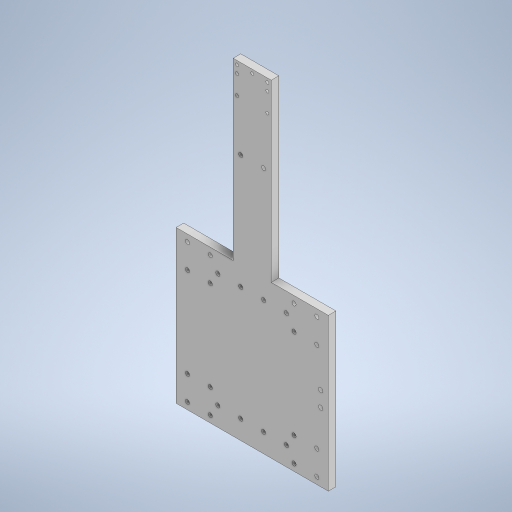
# Autodesk Inventor part: base sotto
Saved by Autodesk Inventor 2024 (Build 280153000, 153)
## iProperties
Created: 2023-12-23
Part Number: base sotto
Material: Generico
Document SubType Name: Modeling
Designer: Giorgio
Density: 1 g/cm^3
Appearance: Default
Mass: 400 g
Surface Area: 880 cm^2
Volume: 400 cm^3
Author: Giorgio
Autodesk Inventor part; units mm, degrees
ref_plane "YZ Plane" through (0, 0, 0) normal (1, 0, 0) x (0, 1, 0)
ref_plane "XZ Plane" through (0, 0, 0) normal (0, 1, 0) x (-1, 0, 0)
ref_plane "XY Plane" through (0, 0, 0) normal (0, 0, 1) x (1, 0, 0)
sketch "Schizzo1" plane through (0, 0, 0) normal (0, 0, 1) x (1, 0, 0)
  line L0 (100, 100) -> (-100, 100)
  line L1 (-100, 100) -> (-100, -100)
  line L2 (-100, -100) -> (100, -100)
  line L3 (100, -100) -> (100, 100)
  line L4 (25, 330) -> (-25, 330)
  line L5 (-25, 330) -> (-25, 100)
  line L6 (-25, 100) -> (25, 100)
  line L7 (25, 100) -> (25, 330)
  circle A0 centre (-20, 325) radius 2
  circle A1 centre (20, 325) radius 2
  circle A2 centre (0, 325) radius 2
  circle A3 centre (85, 91) radius 2.75
  circle A4 centre (85, 59) radius 2.75
  circle A5 centre (55, 91) radius 2.75
  circle A6 centre (55, 59) radius 2.75
  circle A7 centre (85, -59) radius 2.75
  circle A8 centre (-55, -59) radius 2.75
  circle A9 centre (-55, 91) radius 2.75
  circle A10 centre (85, -91) radius 2.75
  circle A11 centre (55, -59) radius 2.75
  circle A12 centre (55, -91) radius 2.75
  circle A13 centre (-85, 91) radius 2.75
  circle A14 centre (-55, 59) radius 2.75
  circle A15 centre (-85, 59) radius 2.75
  circle A16 centre (-85, -59) radius 2.75
  circle A17 centre (-55, -91) radius 2.75
  circle A18 centre (-85, -91) radius 2.75
  circle A19 centre (45, 75) radius 2.75
  circle A20 centre (45, -75) radius 2.75
  circle A21 centre (-45, -75) radius 2.75
  circle A22 centre (-45, 75) radius 2.75
  circle A23 centre (15, 75) radius 2.75
  circle A24 centre (15, -75) radius 2.75
  circle A25 centre (-15, -75) radius 2.75
  circle A26 centre (-15, 75) radius 2.75
  circle A27 centre (15, 225) radius 2.75
  circle A28 centre (-15, 225) radius 2.75
  circle A29 centre (20, 315) radius 2
  circle A30 centre (-20, 315) radius 2
  circle A31 centre (20, 290) radius 2
  circle A32 centre (-20, 290) radius 2
  circle A33 centre (90, 10) radius 3
  circle A34 centre (90, -10) radius 3
  point P0 (0, 0)
  point P1 (25, 100)
  point P2 (0, -100)
  dimension "d0" = 200
  dimension "d1" = 200
  dimension "d4" = 230
  dimension "d5" = 50
  dimension "d6" = 75
  dimension "d7" = 0
  dimension "d8" = 0
  dimension "d9" = 4
  dimension "d10" = 4
  dimension "d11" = 4
  dimension "d12" = 5
  dimension "d13" = 40
  dimension "d14" = 20
  dimension "d15" = 5
  dimension "d16" = 100
  dimension "d17" = 100
  dimension "d18" = 5.5
  dimension "d21" = 32
  dimension "d24" = 30
  dimension "d27" = 5.5
  dimension "d28" = 5.5
  dimension "d29" = 5.5
  dimension "d32" = 32
  dimension "d35" = 30
  dimension "d40" = 30
  dimension "d43" = 32
  dimension "d48" = 30
  dimension "d51" = 32
  dimension "d54" = 150
  dimension "d55" = 59
  dimension "d56" = 150
  dimension "d57" = 59
  dimension "d58" = 15
  dimension "d59" = 15
  dimension "d60" = 15
  dimension "d61" = 15
  dimension "d62" = 5.5
  dimension "d63" = 5.5
  dimension "d64" = 5.5
  dimension "d65" = 5.5
  dimension "d66" = 5.5
  dimension "d67" = 5.5
  dimension "d68" = 5.5
  dimension "d69" = 5.5
  dimension "d70" = 30
  dimension "d71" = 30
  dimension "d72" = 0
  dimension "d73" = 30
  dimension "d74" = 30
  dimension "d75" = 0
  dimension "d76" = 150
  dimension "d77" = 75
  dimension "d79" = 15
  dimension "d80" = 0
  dimension "d81" = 0
  dimension "d82" = 30
  dimension "d83" = 0
  dimension "d84" = 5.5
  dimension "d85" = 5.5
  dimension "d86" = 0
  dimension "d87" = 0
  dimension "d88" = 150
  dimension "d89" = 0
  dimension "d90" = 4
  constraints: 35 centre point, 16 end point, 6 horizontal, 5 vertical, 4 parallel, 2 perpendicular, 1 midpoint, 1 point on line, 26 other
  measures "d0" distance of L2.end L0.start
  measures "d1" distance of L0.start L0.end
  measures "d4" distance of L6.end L4.start
  measures "d5" distance of L4.start L4.end
  measures "d6" distance between parallel lines of L3 L7
  measures "d7" vertical distance of A1.centre A2.centre
  measures "d8" vertical distance of A2.centre A0.centre
  measures "d9" diameter of A0
  measures "d10" diameter of A2
  measures "d11" diameter of A1
  measures "d12" distance from line of L4 A1.centre
  measures "d13" distance of A0.centre A1.centre
  measures "d14" distance of A1.centre A2.centre
  measures "d15" distance from line of L7 A1.centre
  measures "d16" distance from line of L1 point (0, 0)
  measures "d17" distance of point (0, -100) point (0, 0)
  measures "d18" diameter of A3
  measures "d21" distance of A3.centre A4.centre
  measures "d24" distance of A3.centre A5.centre
  measures "d27" diameter of A7
  measures "d28" diameter of A8
  measures "d29" diameter of A9
  measures "d32" distance of A7.centre A10.centre
  measures "d35" distance of A7.centre A11.centre
  measures "d40" distance of A9.centre A13.centre
  measures "d43" distance of A9.centre A14.centre
  measures "d48" distance of A8.centre A16.centre
  measures "d51" distance of A8.centre A17.centre
  measures "d54" distance of A13.centre A16.centre
  measures "d55" vertical distance of A16.centre point (0, 0)
  measures "d56" distance of A3.centre A7.centre
  measures "d57" vertical distance of point (0, 0) A4.centre
  measures "d58" distance from line of L1 A18.centre
  measures "d59" distance from line of L3 A10.centre
  measures "d60" distance from line of L1 A13.centre
  measures "d61" distance from line of L3 A3.centre
  measures "d62" diameter of A19
  measures "d63" diameter of A23
  measures "d64" diameter of A26
  measures "d65" diameter of A22
  measures "d66" diameter of A20
  measures "d67" diameter of A24
  measures "d68" diameter of A25
  measures "d69" diameter of A21
  measures "d70" distance of A23.centre A19.centre
  measures "d71" distance of A22.centre A26.centre
  measures "d72" vertical distance of A26.centre A19.centre
  measures "d73" distance of A24.centre A20.centre
  measures "d74" distance of A21.centre A25.centre
  measures "d75" vertical distance of A24.centre A25.centre
  measures "d76" distance of A19.centre A20.centre
  measures "d77" vertical distance of point (0, 0) A20.centre
  measures "d79" horizontal distance of A24.centre point (0, 0)
  measures "d80" vertical distance of A21.centre A25.centre
  measures "d81" vertical distance of A20.centre A25.centre
  measures "d82" distance of A25.centre A24.centre
  measures "d83" horizontal distance of A26.centre A25.centre
  measures "d84" diameter of A27
  measures "d85" diameter of A28
  measures "d86" vertical distance of A28.centre A27.centre
  measures "d87" horizontal distance of A27.centre A23.centre
  measures "d88" distance of A23.centre A27.centre
  measures "d89" horizontal distance of A28.centre A26.centre
  measures "d90" diameter of A29
extrude "Estrusione1" add sketch "Schizzo1" along normal blind 10
equation "\"d6\" = -0.5 * d5 + 0.5 * d1"
equation "\"d10\" = d9"
equation "\"d11\" = d9"
equation "\"d27\" = d18"
equation "\"d28\" = d18"
equation "\"d29\" = d18"
equation "\"d56\" = d54"
equation "\"d57\" = d55"
equation "\"d59\" = d58"
equation "\"d60\" = d58"
equation "\"d61\" = d58"
equation "\"d63\" = d62"
equation "\"d64\" = d62"
equation "\"d65\" = d62"
equation "\"d66\" = d62"
equation "\"d67\" = d62"
equation "\"d68\" = d62"
equation "\"d69\" = d62"
equation "\"d82\" = 2 * d79"
equation "\"d85\" = d84"
equation "\"d90\" = d9"
